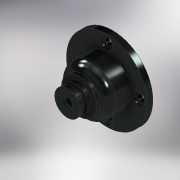
# Autodesk Inventor part: 零件2
Saved by Autodesk Inventor 2020 (Build 240168000, 168)
## iProperties
Created: 2021-04-14
Part Number: 零件2
Material: 灰口铁
Document SubType Name: Modeling
Designer: Luorily
Density: 7.15 g/cm^3
Appearance: 铁灰色 - 抛光
Author: Luorily
Autodesk Inventor part; units mm, degrees
ref_plane "YZ Plane" through (0, 0, 0) normal (1, 0, 0) x (0, 1, 0)
ref_plane "XZ Plane" through (0, 0, 0) normal (0, 1, 0) x (-1, 0, 0)
ref_plane "XY Plane" through (0, 0, 0) normal (0, 0, 1) x (1, 0, 0)
sketch "草图1" plane through (0, 0, 0) normal (1, 0, 0) x (0, 1, 0)
  line L0 (0, 0) -> (13, 0)
  line L1 (13, 0) -> (13, -4)
  line L2 (13, -4) -> (10, -4)
  line L3 (10, -4) -> (10, -8)
  line L4 (10, -8) -> (13, -8)
  line L5 (13, -8) -> (13, -12)
  line L6 (13, -12) -> (18, -12)
  line L7 (18, -12) -> (18, -15)
  line L8 (0, 0) -> (0, -15)
  line L9 (18, -15) -> (25, -15)
  line L10 (0, 0) -> (0, -46)
  line L11 (0, -46) -> (41, -46)
  line L12 (41, -46) -> (41, -40)
  line L13 (41, -40) -> (25, -40)
  line L14 (25, -40) -> (25, -15)
  dimension "d0" = 13
  dimension "d1" = 4
  dimension "d2" = 3
  dimension "d3" = 4
  dimension "d4" = 3
  dimension "d5" = 4
  dimension "d6" = 5
  dimension "d7" = 3
  dimension "d8" = 25
  dimension "d9" = 46
  dimension "d10" = 41
  dimension "d11" = 6
  dimension "d12" = 16
  constraints: 30 end point, 9 perpendicular, 2 point on line, 2 vertical, 1 horizontal
  measures "d0" distance of L0.start L0.end
  measures "d1" distance of L0.end L1.end
  measures "d2" distance of L1.end L2.end
  measures "d3" distance of L2.end L3.end
  measures "d4" distance of L3.end L4.end
  measures "d5" distance of L4.end L5.end
  measures "d6" distance of L5.end L6.end
  measures "d7" distance of L7.end L6.end
  measures "d8" distance of L8.end L9.end
  measures "d9" distance of L0.start L10.end
  measures "d10" distance of L10.end L11.end
  measures "d11" distance of L11.end L12.end
  measures "d12" distance of L12.end L13.end
revolve "旋转1" add sketch "草图1" angle 360 about axis through (0, 0, 0) along (0, 0, -1)
sketch "草图2" plane through (0, 0, 0) normal (0, 0, 1) x (1, 0, 0)
  circle A0 centre (0, 0) radius 13 projected
  constraints: 1 coincident
hole "孔1" at (0, 0, 0) direction (0, 0, -1) diameter 8.376 end through all thread size "M10x1.5" designation "M10" class "6H" standard "GB Metric profile"
sketch "草图3" plane through (0, 0, -46) normal (0, 0, -1) x (-1, 0, 0)
  circle A0 centre (0, 0) radius 4.188 projected
  circle A1 centre (0, 0) radius 41 projected
  circle A2 centre (0, 0) radius 20
  dimension "d21" = 40
  constraints: 1 centre point, 1 coincident
  measures "d21" diameter of A2
extrude "拉伸1" cut sketch "草图3" against normal blind 26 contours A2
fillet "圆角1" radius 5 1 edges at (20, 0, -20)
fillet "圆角2" radius 10 1 edges at (0, -25, -15)
sketch "草图4" plane through (0, 0, -40) normal (0, 0, 1) x (1, 0, 0)
  circle A0 centre (0, 0) radius 41 projected
  circle A1 centre (0, 0) radius 33
  point P0 (-33, 0)
  dimension "d26" = 66
  constraints: 1 coincident, 1 horizontal alignment, 2 other
hole "孔2" at (-33, 0, -40) direction (0, 0, -1) diameter 7 end through all
sketch "草图5" plane through (0, 0, -40) normal (0, 0, 1) x (1, 0, 0)
  circle A0 centre (-33, 0) radius 3.5 projected
  point P0 (0, 0)
  constraints: 1 coincident
hole "孔3" at (-33, 0, -40) direction (0, 0, -1) diameter 12 depth 2
pattern_circular "环形阵列1" count 4 over 360 about axis through (0, 0, -124.7558) along (0, 0, 1) of "孔3", "孔2"
chamfer "倒角1" distance 1 angle 45 1 edges at (0, 4.188, 0)
